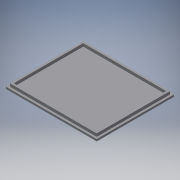
# Autodesk Inventor part: Arduino SMB-BNC box lid
Saved by Autodesk Inventor 2016 (Build 200138000, 138)
## iProperties
Created: 2013-05-02
Part Number: Arduino SMB-BNC box lid
Material: Generic
Document SubType Name: Modeling
Designer: kthorn
Density: 1 g/cm^3
Appearance: Default
Author: kthorn
Autodesk Inventor part; units mm, degrees
ref_plane "YZ Plane" through (0, 0, 0) normal (1, 0, 0) x (0, 1, 0)
ref_plane "XZ Plane" through (0, 0, 0) normal (0, 1, 0) x (-1, 0, 0)
ref_plane "XY Plane" through (0, 0, 0) normal (0, 0, 1) x (1, 0, 0)
sketch "Sketch1" plane through (0, 0, 0) normal (0, 0, 1) x (1, 0, 0)
  line L0 (-7.7165, 5.0063) -> (84.5835, 5.0063)
  line L1 (84.5835, 5.0063) -> (84.5835, -73.5937)
  line L2 (84.5835, -73.5937) -> (-7.7165, -73.5937)
  line L3 (-7.7165, -73.5937) -> (-7.7165, 5.0063)
  point P0 (0, 0)
  dimension "d0" = 92.3
  dimension "d1" = 78.6
  constraints: 8 end point, 2 parallel, 1 horizontal, 1 perpendicular
  measures "d0" distance of L0.start L0.end
  measures "d1" distance of L2.end L0.start
extrude "Extrusion1" add sketch "Sketch1" along normal blind 2
sketch "Sketch2" plane through (0, 0, 2) normal (0, 0, 1) x (1, 0, 0)
  line L0 (84.5835, 5.0063) -> (-7.7165, 5.0063) projected
  line L1 (-7.7165, 5.0063) -> (-7.7165, -73.5937) projected
  line L2 (-7.7165, -73.5937) -> (84.5835, -73.5937) projected
  line L3 (84.5835, -73.5937) -> (84.5835, 5.0063) projected
  line L4 (-5.7165, 3.0063) -> (82.5835, 3.0063)
  line L5 (82.5835, 3.0063) -> (82.5835, -71.5937)
  line L6 (82.5835, -71.5937) -> (-5.7165, -71.5937)
  line L7 (-5.7165, -71.5937) -> (-5.7165, 3.0063)
  line L8 (-3.7165, 1.0063) -> (80.5835, 1.0063)
  line L9 (80.5835, 1.0063) -> (80.5835, -69.5937)
  line L10 (80.5835, -69.5937) -> (-3.7165, -69.5937)
  line L11 (-3.7165, -69.5937) -> (-3.7165, 1.0063)
  line L12 (38.4335, 3.0063) -> (38.4335, 1.0063) construction
  line L13 (80.5835, -29.2) -> (82.5835, -29.2) construction
  line L14 (71.1302, 3.0063) -> (71.1302, 5.0063) construction
  line L15 (82.5835, -16.3714) -> (84.5835, -16.3714) construction
  line L16 (11.0323, -71.5937) -> (11.0323, -73.5937) construction
  line L17 (-5.7165, -42.5946) -> (-7.7165, -42.5946) construction
  line L18 (31.7844, -69.5937) -> (31.7844, -71.5937) construction
  line L19 (-3.7165, -29.2) -> (-5.7165, -29.2) construction
  point P0 (0, 0)
  dimension "d4" = 2
  dimension "d5" = 2
  constraints: 32 end point, 14 point on line, 10 perpendicular, 6 equal length, 4 parallel, 2 horizontal, 2 midpoint
  measures "d4" distance of L17.start L17.end
  measures "d5" distance of L13.start L13.end
extrude "Extrusion2" add sketch "Sketch2" along normal blind 3 contours L4 L5 L6 L7
body "Solid1"
